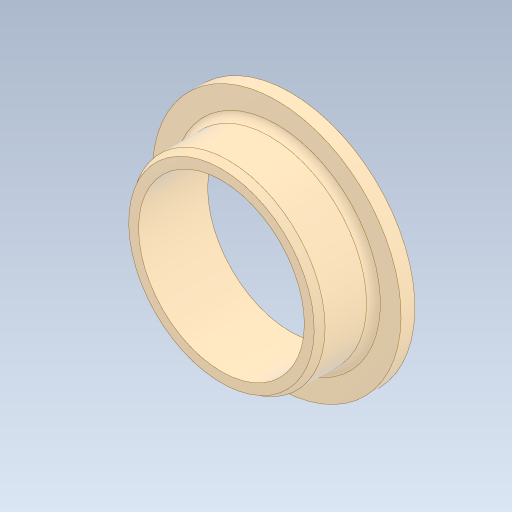
# Autodesk Inventor part: _GFM-0608-04
Saved by Autodesk Inventor 2024 (Build 280153000, 153)
## iProperties
Created: 2023-09-16
Part Number: _GFM-0608-04
Material: アセタール樹脂、黒
Document SubType Name: Modeling
Designer: michi
Density: 1.425 g/cm^3
Appearance: 滑らか - オフホワイト
Author: michi
Autodesk Inventor part; units mm, degrees
ref_plane "YZ Plane" through (0, 0, 0) normal (1, 0, 0) x (0, 1, 0)
ref_plane "XZ Plane" through (0, 0, 0) normal (0, 1, 0) x (-1, 0, 0)
ref_plane "XY Plane" through (0, 0, 0) normal (0, 0, 1) x (1, 0, 0)
sketch "スケッチ1" plane through (0, 0, 0) normal (1, 0, 0) x (0, 1, 0)
  line L0 (0, -1) -> (0, 6) construction
  line L1 (6, 5) -> (7, 5)
  line L2 (7, 5) -> (7, 0)
  line L3 (7, 0) -> (6, 0)
  line L4 (6, 0) -> (6, 5)
  line L5 (7, 1) -> (9, 1)
  line L6 (9, 1) -> (9, 0)
  line L7 (9, 0) -> (7, 0)
  line L8 (7, 0) -> (7, 1)
  point P0 (0, 0)
  point P1 (7, 0)
  dimension "d0" = 12
  dimension "d1" = 14
  dimension "d10" = 5
  dimension "d14" = 1
  dimension "d15" = 18
  constraints: 16 end point, 4 parallel, 2 collinear, 2 horizontal, 2 perpendicular, 1 point on line
  measures "d0" diameter of L4 L0
  measures "d1" diameter of L2 L0
  measures "d10" distance of L1.end L2.end
  measures "d14" distance of L5.end L6.end
  measures "d15" diameter of L6 L0
revolve "回転1" add sketch "スケッチ1" angle 360 about axis through (0, 0, -10) along (0, 0, 1)
chamfer "面取り1" distance 0.5 angle 30 1 edges at (0, -7, 5) measured on face at (0.5633, 6.9773, 2.3333)
fillet "フィレット2" radius 0.5 1 edges at (0, -7, 1)
